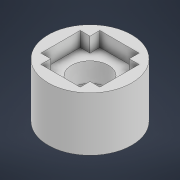
# Autodesk Inventor part: Zahnrad_außen
Saved by Autodesk Inventor 2021 (Build 250183000, 183)
## iProperties
Created: 2021-01-01
Part Number: Zahnrad_außen
Material: Generisch
Document SubType Name: Modeling
Designer: laure
Density: 1 g/cm^3
Appearance: Vorgabe
Author: laure
## iProperties of the stored document _3D-Druck.ipt
Created: 2021-01-01
Part Number: _3D-Druck
Material: Generisch
Document SubType Name: Modeling
Designer: laure
Density: 1 g/cm^3
Appearance: Vorgabe
Author: laure
Autodesk Inventor part; units mm, degrees
ref_plane "YZ Plane" through (0, 0, 0) normal (1, 0, 0) x (0, 1, 0)
ref_plane "XZ Plane" through (0, 0, 0) normal (0, 1, 0) x (-1, 0, 0)
ref_plane "XY Plane" through (0, 0, 0) normal (0, 0, 1) x (1, 0, 0)
sketch "Skizze1" plane through (0, 0, 0) normal (0, 1, 0) x (-1, 0, 0)
  circle A0 centre (0, 0) radius 8.5
  line L0 (0, -11.9) -> (0, 11.9) projected
  line L1 (11.9, 0) -> (-11.9, 0) projected
  line L2 (6, -6) -> (-6, -6)
  line L3 (-6, -6) -> (-6, 6)
  line L4 (6, 6) -> (6, -6)
  line L5 (6, -6) -> (-6, 6) construction
  line L6 (-6, -6) -> (6, 6) construction
  line L7 (6, 6) -> (-6, 6)
  point P0 (6, -1)
  point P1 (-6, -1)
  dimension "d10" = 12
  dimension "d12" = 17
  dimension "d53" = 12
  constraints: 12 end point, 2 horizontal, 2 midpoint, 2 point on line, 1 centre point, 1 parallel, 1 perpendicular, 2 other
  measures "d10" distance of L3.end L4.start
  measures "d12" diameter of A0
  measures "d53" distance between parallel lines of L7 L2
extrude "Extrusion1" add sketch "Skizze1" along normal blind 6
sketch "Skizze3" plane through (0, 0, 0) normal (0, -1, 0) x (1, 0, 0)
  circle A0 centre (0, 0) radius 8.5
  dimension "d99" = 17
  constraints: 1 centre point, 1 coincident
  measures "d99" diameter of A0
extrude "Extrusion3" add sketch "Skizze3" along normal blind 6
sketch "Skizze9" plane through (0, 6, 0) normal (0, 1, 0) x (1, 0, 0)
  line L0 (-6, 6) -> (6, 6)
  line L1 (6, 6) -> (6, -6)
  line L2 (6, -6) -> (-6, -6)
  line L3 (-6, -6) -> (-6, 6)
  line L4 (-6, 6) -> (6, -6) construction
  line L5 (6, 6) -> (-6, -6) construction
  point P0 (0, 0)
  dimension "d54" = 12
  dimension "d55" = 12
  constraints: 12 end point, 2 midpoint, 2 parallel, 1 horizontal, 1 perpendicular
  measures "d54" distance of L1.end L2.end
  measures "d55" distance of L0.end L1.end
extrude "Extrusion9" cut sketch "Skizze9" against normal blind 6
sketch "Skizze10" plane through (0, 0, 0) normal (0, 1, 0) x (1, 0, 0)
  circle A0 centre (0, 0) radius 3.75
  dimension "d58" = 7.5
  constraints: 1 centre point, 1 coincident
  measures "d58" diameter of A0
extrude "Extrusion10" cut sketch "Skizze10" against normal blind 4
sketch "Skizze12" plane through (0, 6, 0) normal (0, 1, 0) x (1, 0, 0)
  line L0 (-6, 6) -> (-4, 6)
  line L1 (-4, 6) -> (-4, 4)
  line L2 (-4, 4) -> (-6, 4)
  line L3 (-6, 4) -> (-6, 6)
  line L4 (6, 6) -> (6, -6) projected
  line L5 (6, 6) -> (4, 6)
  line L6 (4, 6) -> (4, 4)
  line L7 (4, 4) -> (6, 4)
  line L8 (6, 4) -> (6, 6)
  line L9 (6, -6) -> (-6, -6) projected
  line L10 (-6, -6) -> (-4, -6)
  line L11 (-4, -6) -> (-4, -4)
  line L12 (-4, -4) -> (-6, -4)
  line L13 (-6, -4) -> (-6, -6)
  line L14 (6, -6) -> (4, -6)
  line L15 (4, -6) -> (4, -4)
  line L16 (4, -4) -> (6, -4)
  line L17 (6, -4) -> (6, -6)
  point P0 (0, 0)
  dimension "d64" = 2
  dimension "d65" = 2
  dimension "d66" = 2
  dimension "d67" = 2
  dimension "d68" = 2
  dimension "d69" = 2
  dimension "d70" = 2
  dimension "d71" = 2
  constraints: 32 end point, 8 parallel, 4 horizontal, 4 perpendicular
  measures "d64" distance of L1.end L2.end
  measures "d65" distance of L0.end L1.end
  measures "d66" distance of L7.end L6.end
  measures "d67" distance between parallel lines of L7 L5
  measures "d68" distance of L12.end L11.end
  measures "d69" distance of L11.end L10.end
  measures "d70" distance of L15.end L16.end
  measures "d71" distance of L14.end L15.end
extrude "Extrusion12" add sketch "Skizze12" against normal up to surface (6 mm away)
sketch "Skizze13" plane through (0, -6, 0) normal (0, -1, 0) x (1, 0, 0)
  line L0 (-2.5, 5.5) -> (2.5, 5.5)
  line L1 (5.5, 2.5) -> (5.5, -2.5)
  line L2 (2.5, -5.5) -> (-2.5, -5.5)
  line L3 (-5.5, -2.5) -> (-5.5, 2.5)
  line L4 (0, 12.6) -> (0, -12.6) projected
  line L5 (-12.6, 0) -> (12.6, 0) projected
  line L6 (2.5, 5.5) -> (2.5, 2.5)
  line L7 (2.5, 2.5) -> (5.5, 2.5)
  line L8 (-2.5, 5.5) -> (-2.5, 2.5)
  line L9 (-2.5, 2.5) -> (-5.5, 2.5)
  line L10 (-2.5, -5.5) -> (-2.5, -2.5)
  line L11 (-2.5, -2.5) -> (-5.5, -2.5)
  line L12 (2.5, -5.5) -> (2.5, -2.5)
  line L13 (2.5, -2.5) -> (5.5, -2.5)
  circle A0 centre (0, 0) radius 8.5
  dimension "d76" = 3
  dimension "d77" = 3
  dimension "d78" = 3
  dimension "d79" = 3
  dimension "d80" = 3
  dimension "d81" = 3
  dimension "d82" = 3
  dimension "d83" = 3
  dimension "d84" = 90
  dimension "d85" = 2.5
  dimension "d86" = 2.5
  dimension "d87" = 2.5
  dimension "d88" = 2.5
  dimension "d89" = 90
  dimension "d90" = 17
  constraints: 24 end point, 2 parallel, 1 centre point, 1 coincident, 1 horizontal, 1 perpendicular, 2 other
  measures "d76" distance of L1.start L6.end
  measures "d77" distance of L0.end L6.end
  measures "d78" distance of L3.end L8.end
  measures "d79" distance of L0.start L8.end
  measures "d80" distance of L3.start L10.end
  measures "d81" distance of L2.end L10.end
  measures "d82" distance of L1.end L12.end
  measures "d83" distance of L2.start L12.end
  measures "d84" angle of L4 L7
  measures "d85" distance between parallel lines of L4 L12
  measures "d86" distance between parallel lines of L5 L13
  measures "d87" distance between parallel lines of L4 L10
  measures "d88" distance between parallel lines of L5 L9
  measures "d89" angle of L5 L6
  measures "d90" diameter of A0
extrude "Extrusion13" add sketch "Skizze13" along normal blind 2 contours L8 L9 L3 L5 A0 L4 L0 | L4 A0 L5 L1 L7 L6 L0 | A0 L4 L2 L12 L13 L1 L5 | L5 L3 L11 L10 L2 L4 A0
sketch "Skizze14" plane through (0, -4, 0) normal (0, 1, 0) x (1, 0, 0)
  circle A0 centre (0, 0) radius 1.6
  dimension "d93" = 3.2
  constraints: 1 centre point, 1 coincident
  measures "d93" diameter of A0
extrude "Extrusion14" cut sketch "Skizze14" against normal up to surface (2 mm away)
sketch "Skizze15" plane through (0, 6, 0) normal (0, 1, 0) x (1, 0, 0)
  circle A0 centre (0, 0) radius 9
  line L0 (-4, 6) -> (4, 6) projected
  line L1 (-4, 6) -> (4, 6)
  line L2 (4, 4) -> (6, 4) projected
  line L3 (4, 6) -> (4, 4)
  line L4 (6, 4) -> (6, -4) projected
  line L5 (4, 4) -> (6, 4)
  line L6 (6, 4) -> (6, -4)
  line L7 (6, -4) -> (4, -4)
  line L8 (4, -4) -> (4, -6) projected
  line L9 (4, -4) -> (4, -6)
  line L10 (4, -6) -> (-4, -6) projected
  line L11 (4, -6) -> (-4, -6)
  line L12 (-4, -4) -> (-4, -6) projected
  line L13 (-4, -6) -> (-4, -4)
  line L14 (-6, -4) -> (-4, -4) projected
  line L15 (-4, -4) -> (-6, -4)
  line L16 (-4, 4) -> (-6, 4) projected
  line L17 (-6, -4) -> (-6, 4)
  line L18 (-6, 4) -> (-4, 4)
  line L19 (-4, 4) -> (-4, 6) projected
  line L20 (-4, 4) -> (-4, 6)
  dimension "d96" = 18
  constraints: 24 end point, 8 perpendicular, 4 collinear, 1 centre point, 1 coincident, 1 point on line
  measures "d96" diameter of A0
extrude "Extrusion15" cut sketch "Skizze15" against normal blind 3
